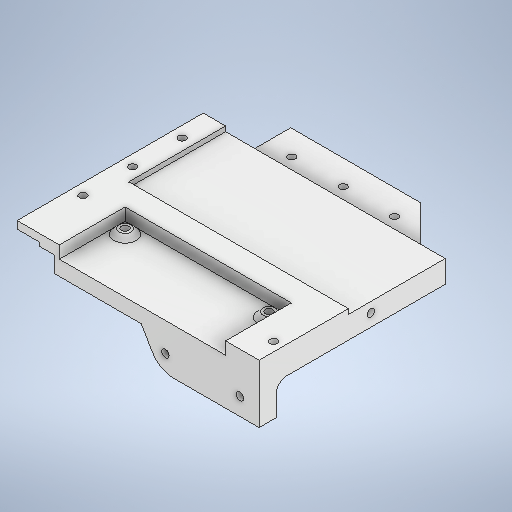
# Autodesk Inventor part: BottomSlideMountExtension
Saved by Autodesk Inventor 2026.2 (Build 302298000, 298)
## iProperties
Created: 2026-04-01
Part Number: BottomSlideMountExtension
Material: ABS Plastic
Document SubType Name: Modeling
Designer: gaoet
Density: 1.06 g/cm^3
Appearance: Smooth - White
Author: gaoet
Autodesk Inventor part; units mm, degrees
ref_plane "YZ Plane" through (0, 0, 0) normal (1, 0, 0) x (0, 1, 0)
ref_plane "XZ Plane" through (0, 0, 0) normal (0, 1, 0) x (-1, 0, 0)
ref_plane "XY Plane" through (0, 0, 0) normal (0, 0, 1) x (1, 0, 0)
sketch "Sketch1" plane through (0, 0, 0) normal (0, 0, 1) x (1, 0, 0)
  line L0 (-48.75, -5.5) -> (48.75, -5.5)
  line L1 (48.75, -5.5) -> (48.75, 5.5)
  line L2 (48.75, 5.5) -> (-48.75, 5.5)
  line L3 (-48.75, 5.5) -> (-48.75, -5.5)
  line L4 (-48.75, -5.5) -> (48.75, 5.5) construction
  line L5 (48.75, -5.5) -> (-48.75, 5.5) construction
  line L6 (-48.75, 2.5) -> (-39.75, 2.5)
  line L7 (-39.75, 2.5) -> (-39.75, 1)
  line L8 (-39.75, 1) -> (-33.5, 1)
  line L9 (-33.5, 1) -> (-33.5, -5.5)
  point P0 (0, 0)
  dimension "d0" = 11
  dimension "d1" = 97.5
  dimension "d2" = 9
  dimension "d3" = 6.25
  dimension "d4" = 1.5
  dimension "d5" = 6.5
  constraints: 20 end point, 3 perpendicular, 2 horizontal, 2 midpoint, 2 parallel, 2 point on line, 1 vertical
  measures "d0" distance of L0.end L1.end
  measures "d1" distance of L1.end L2.end
  measures "d2" distance of L6.start L6.end
  measures "d3" distance of L7.end L8.end
  measures "d4" distance of L6.end L7.end
  measures "d5" distance of L8.end L9.end
extrude "Extrusion1" add sketch "Sketch1" along normal blind 75 contours L9 L8 L7 L6 L3 L2 L1 L0
sketch "Sketch2" plane through (-48.75, 2.5, 0) normal (0, -1, 0) x (1, 0, 0)
  line L0 (0, 0) -> (9, 0) projected
  point P0 (48.75, 0)
  point P1 (4.5, 13)
  point P2 (4.5, 33)
  point P3 (4.5, 53)
  point P4 (4.5, 0)
  point P5 (4.5, 0)
  point P6 (4.5, 73)
  dimension "d8" = 13
  dimension "d9" = 20
  dimension "d10" = 20
  dimension "d11" = 20
  constraints: 4 vertical alignment, 2 midpoint
  measures "d8" distance of point (4.5, 0) point (4.5, 13)
  measures "d9" distance of point (4.5, 13) point (4.5, 33)
  measures "d10" distance of point (4.5, 53) point (4.5, 33)
  measures "d11" distance of point (4.5, 53) point (4.5, 73)
hole "Hole1" at (-44.25, 2.5, 13) at (-44.25, 2.5, 33) at (-44.25, 2.5, 53) direction (0, 1, 0) diameter 3 depth 15
sketch "Sketch3" plane through (48.75, -5.5, 0) normal (1, 0, 0) x (0, 0, -1)
  line L0 (0, 0) -> (0, 11) projected
  line L1 (0, 11) -> (-75, 11) projected
  line L2 (-75, 0) -> (-75, 11) projected
  line L3 (0, 0) -> (-75, 0) projected
  point P0 (0, 5.5)
  point P1 (-30, 5)
  point P2 (0, 5.5)
  dimension "d19" = 30
  dimension "d20" = 5
  constraints: 1 midpoint
  measures "d19" horizontal distance of point (0, 5.5) point (-30, 5)
  measures "d20" distance from line of L3 point (-30, 5)
hole "Hole2" at (48.75, -0.5, 30) direction (-1, 0, 0) diameter 3 depth 15
sketch "Sketch4" plane through (-33.5, -5.5, 0) normal (0, -1, 0) x (1, 0, 0)
  line L0 (0, 0) -> (82.25, 0) projected
  line L1 (82.25, 0) -> (82.25, 75) projected
  line L2 (0, 75) -> (82.25, 75) projected
  line L3 (0, 0) -> (0, 75) projected
  line L4 (0, 0) -> (0, -20)
  line L5 (0, -20) -> (62.25, -20)
  line L6 (62.25, -20) -> (62.25, 0)
  point P0 (33.5, 0)
  dimension "d28" = 20
  dimension "d29" = 20
  constraints: 6 end point, 2 perpendicular, 1 point on line, 1 vertical
  measures "d28" distance of L5.end L6.end
  measures "d29" distance between parallel lines of L1 L6
extrude "Extrusion2" add sketch "Sketch4" against normal blind 3.5 contours L0 L6 L5 L4
chamfer "Chamfer1" distance 10 angle 45 2 edges at (28.75, -3.75, -20) (28.75, -3.75, 0)
sketch "Sketch5" plane through (-33.5, -5.5, 75) normal (0, -1, 0) x (1, 0, 0)
  line L0 (0, -95) -> (0, 0) projected
  line L1 (0, -95) -> (52.25, -95) projected
  line L2 (62.25, -75) -> (0, -75) projected
  line L3 (62.25, -75) -> (62.25, -95)
  line L4 (62.25, -95) -> (52.25, -95)
  point P0 (33.5, -75)
  point P1 (10.375, -85)
  point P2 (31.125, -85)
  point P3 (51.875, -85)
  dimension "d36" = 10.375
  dimension "d37" = 20.75
  dimension "d38" = 20.75
  dimension "d39" = 20
  dimension "d40" = 10
  constraints: 4 end point, 2 horizontal alignment, 1 perpendicular, 1 vertical
  measures "d36" distance from line of L0 point (10.375, -85)
  measures "d37" distance of point (31.125, -85) point (10.375, -85)
  measures "d38" distance of point (51.875, -85) point (31.125, -85)
  measures "d39" distance between parallel lines of L1 L2
  measures "d40" distance from line of point (10.375, -85) L2
hole "Hole3" at (-23.125, -5.5, -10) at (-2.375, -5.5, -10) at (18.375, -5.5, -10) direction (0, 1, 0) diameter 3 depth 15
sketch "Sketch6" plane through (0, 0, 75) normal (0, 0, 1) x (1, 0, 0)
  line L0 (-33.5, -5.5) -> (48.75, -5.5) projected
  line L1 (48.75, -5.5) -> (48.75, -18)
  line L2 (48.75, -18) -> (8.5, -18)
  line L3 (8.5, -18) -> (-56.5, 94.5833)
  line L4 (-56.5, 94.5833) -> (-56.5, 62)
  point P0 (0, 0)
  point P1 (48.75, -11.75)
  point P2 (1.2831, -5.5)
  dimension "d48" = 12.5
  dimension "d49" = 120
  dimension "d50" = 105.25
  dimension "d51" = 80
  dimension "d52" = 65
  constraints: 8 end point, 2 point on line, 2 vertical, 1 horizontal, 1 midpoint
  measures "d48" distance between parallel lines of L0 L2
  measures "d49" angle of L2 L3
  measures "d50" distance from line of point (48.75, -11.75) L4
  measures "d51" distance from line of L4.end L2
  measures "d52" distance from line of L4 L2.end
extrude "Extrusion3" add sketch "Sketch6" against normal blind 7
fillet "Fillet1" radius 4 1 edges at (25.0166, -5.5, 68)
fillet "Fillet2" radius 10 1 edges at (8.5, -18, 71.5)
sketch "Sketch7" plane through (0, 0, 75) normal (0, 0, 1) x (1, 0, 0)
  arc A0 (5.6132, -13) -> (14.2735, -18) centre (14.2735, -8) ccw projected
  line L0 (14.2735, -18) -> (48.75, -18) projected
  line L1 (48.75, -18) -> (48.75, 5.5) projected
  line L2 (48.75, 5.5) -> (-48.75, 5.5) projected
  line L3 (-48.75, 5.5) -> (-48.75, 2.5) projected
  line L4 (-48.75, 2.5) -> (-39.75, 2.5) projected
  line L5 (-39.75, 2.5) -> (-39.75, 1) projected
  line L6 (-39.75, 1) -> (-33.5, 1) projected
  line L7 (-33.5, 1) -> (-33.5, -5.5) projected
  line L8 (-33.5, -5.5) -> (1.2831, -5.5) projected
  line L9 (1.2831, -5.5) -> (5.6132, -13) projected
  point P0 (0, 0)
  point P1 (41, -11)
  point P2 (11, -11)
  dimension "d57" = 30
  dimension "d58" = 7.75
  dimension "d59" = 7
  constraints: 1 horizontal alignment
  measures "d57" distance of point (41, -11) point (11, -11)
  measures "d58" distance from line of L1 point (41, -11)
  measures "d59" distance from line of L0 point (41, -11)
hole "Hole4" at (41, -11, 75) at (11, -11, 75) direction (0, 0, -1) diameter 3 depth 15
sketch "Sketch8" plane through (-48.75, 5.5, 0) normal (0, 1, 0) x (1, 0, 0)
  line L0 (97.5, -75) -> (0, -75) projected
  line L1 (97.5, 0) -> (97.5, -75) projected
  point P0 (48.75, 0)
  point P1 (93.875, -65.5)
  dimension "d67" = 9.5
  dimension "d68" = 3.625
  measures "d67" distance from line of L0 point (93.875, -65.5)
  measures "d68" distance from line of L1 point (93.875, -65.5)
hole "Hole5" at (45.125, 5.5, 65.5) direction (0, -1, 0) diameter 3 depth 10
sketch "Sketch9" plane through (-48.75, 5.5, 0) normal (0, 1, 0) x (1, 0, 0)
  line L0 (18, -79.5) -> (83, -79.5)
  line L1 (83, -79.5) -> (83, -49.5)
  line L2 (83, -49.5) -> (18, -49.5)
  line L3 (18, -49.5) -> (18, -79.5)
  line L4 (18, -79.5) -> (83, -49.5) construction
  line L5 (83, -79.5) -> (18, -49.5) construction
  line L6 (21.5, -76) -> (79.5, -76)
  line L7 (79.5, -76) -> (79.5, -53)
  line L8 (79.5, -53) -> (21.5, -53)
  line L9 (21.5, -53) -> (21.5, -76)
  line L10 (21.5, -76) -> (79.5, -53) construction
  line L11 (79.5, -76) -> (21.5, -53) construction
  line L12 (97.5, -75) -> (0, -75) projected
  line L13 (97.5, 0) -> (97.5, -75) projected
  line L14 (17, -48.5) -> (84, -48.5)
  line L15 (84, -48.5) -> (84, -80.5)
  line L16 (84, -80.5) -> (17, -80.5)
  line L17 (17, -80.5) -> (17, -48.5)
  point P0 (48.75, 0)
  point P1 (50.5, -64.5)
  point P2 (83, -75)
  point P3 (84, -75)
  point P4 (17, -75)
  point P5 (18, -75)
  dimension "d76" = 65
  dimension "d77" = 30
  dimension "d78" = 58
  dimension "d79" = 23
  dimension "d80" = 47
  dimension "d97" = 4.5
  dimension "d103" = 1
  constraints: 32 end point, 6 parallel, 4 midpoint, 3 perpendicular, 2 horizontal, 3 other
  measures "d76" distance of L2.end L1.end
  measures "d77" distance between parallel lines of L0 L2
  measures "d78" distance of L8.end L7.end
  measures "d79" distance of L7.end L6.end
  measures "d80" distance from line of L13 point (50.5, -64.5)
  measures "d97" distance between parallel lines of L12 L0
  measures "d103" distance between parallel lines of L2 L14
extrude "Extrusion4" cut sketch "Sketch9" against normal blind 5 contours L3 L12 L9 L6 L7 L1 L0 | L12 L17 L14 L15 L1 L2 L3 | L3 L2 L1 L12 L7 L8 L9 | L12 L7 L6 L9 | L9 L8 L7 L12
hole "Hole6" at (30.75, 5.5, 53) at (-27.25, 5.5, 53) direction (0, -1, 0) diameter 3 depth 10
sketch "Sketch10" plane through (-48.75, 0.5, 0) normal (0, 1, 0) x (1, 0, 0)
  circle A0 centre (21.5, -53) radius 1.5 projected
  circle A1 centre (79.5, -53) radius 1.5 projected
  line L0 (84, -75) -> (17, -75) projected
  circle A2 centre (21.5, -53) radius 2.5
  circle A3 centre (79.5, -53) radius 2.5
  circle A4 centre (76.5, -76) radius 2.5
  circle A5 centre (18.5, -76) radius 2.5
  line L1 (84, -48.5) -> (84, -75) projected
  line L2 (17, -48.5) -> (84, -48.5) projected
  line L3 (17, -75) -> (17, -48.5) projected
  point P0 (48.75, 0)
  point P1 (78.7913, -75)
  point P2 (74.2087, -75)
  point P3 (20.7913, -75)
  point P4 (20.7913, -75)
  dimension "d91" = 1
  constraints: 4 centre point, 3 equal radius, 1 coincident
  measures "d91" radial gap between concentric circles of A0 A2
extrude "Extrusion5" add sketch "Sketch10" along normal blind 2 contours A2 | A3
chamfer "Chamfer2" distance 2 angle 45 2 edges at (28.25, 0.5, 53) (-29.75, 0.5, 53)
sketch "Sketch11" plane through (-48.75, 5.5, 0) normal (0, 1, 0) x (1, 0, 0)
  line L0 (97.5, -75) -> (84, -75) projected
  line L1 (97.5, 0) -> (97.5, -75) projected
  line L2 (97.5, 0) -> (0, 0) projected
  line L3 (0, 0) -> (0, -75) projected
  line L4 (17, -75) -> (0, -75) projected
  circle A0 centre (93.875, -65.5) radius 1.5 projected
  circle A1 centre (4.5, -53) radius 1.5 projected
  circle A2 centre (4.5, -33) radius 1.5 projected
  circle A3 centre (4.5, -13) radius 1.5 projected
  line L5 (9, 0.062) -> (9, -75.3378)
  line L6 (0, -39) -> (97.5, -39)
  line L7 (84, -48.5) -> (84, -75) projected
  line L8 (17, -75) -> (17, -48.5) projected
  line L9 (17, -48.5) -> (84, -48.5) projected
  point P0 (48.75, 0)
  point P1 (90.75, -75)
  point P2 (9, -39)
  point P3 (9, 0)
  dimension "d99" = 9
  dimension "d100" = 36
  constraints: 4 end point, 2 point on line, 1 horizontal, 1 midpoint, 1 vertical
  measures "d99" distance between parallel lines of L3 L5
  measures "d100" distance from line of point (90.75, -75) L6
extrude "Extrusion6" cut sketch "Sketch11" against normal blind 2 contours L6 L5 L2 L1
equation "\"d10\" = d9"
equation "\"d11\" = d10"
equation "\"d36\" = 0.166667 * d35"
equation "\"d37\" = 2 * d36"
equation "\"d38\" = d37"
equation "\"d40\" = 0.5 * d39"
equation "\"d35\" = 62.25"
body "Solid1"
